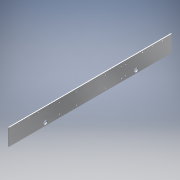
# Autodesk Inventor part: Bumper Plate
Saved by Autodesk Inventor 2019 (Build 230136000, 136)
## iProperties
Created: 2019-10-20
Part Number: Bumper Plate
Material: Aluminum 6061
Document SubType Name: Modeling
Designer: admin
Density: 2.7 g/cm^3
Appearance: Aluminum - Flat
Mass: 1233.5 g
Surface Area: 1935.72 cm^2
Volume: 456.852 cm^3
Author: admin
Autodesk Inventor part; units mm, degrees
ref_plane "YZ Plane" through (0, 0, 0) normal (1, 0, 0) x (0, 1, 0)
ref_plane "XZ Plane" through (0, 0, 0) normal (0, 1, 0) x (-1, 0, 0)
ref_plane "XY Plane" through (0, 0, 0) normal (0, 0, 1) x (1, 0, 0)
sketch "Sketch1" plane through (0, 0, 0) normal (1, 0, 0) x (0, 1, 0)
  line L0 (-50, 489.5) -> (50, 489.5)
  line L1 (50, 489.5) -> (50, -489.5)
  line L2 (50, -489.5) -> (-50, -489.5)
  line L3 (-50, -489.5) -> (-50, 489.5)
  line L4 (-50, 489.5) -> (50, -489.5) construction
  line L5 (50, 489.5) -> (-50, -489.5) construction
  point P0 (0, 0)
  dimension "d0" = 979
  dimension "d1" = 100
  constraints: 12 end point, 2 midpoint, 2 parallel, 1 horizontal, 1 perpendicular
  measures "d0" distance of L0.end L1.end
  measures "d1" distance of L0.start L0.end
extrude "Extrusion1" add sketch "Sketch1" along normal blind 5
sketch "Sketch2" plane through (5, 0, 0) normal (1, 0, 0) x (0, 0, -1)
  circle A0 centre (-270.411, -31.452) radius 12.25
  line L0 (-489.5, -50) -> (489.5, -50) projected
  line L1 (-489.5, 50) -> (-489.5, -50) projected
  circle A1 centre (274.562, -31.452) radius 12.25
  line L2 (489.5, -50) -> (489.5, 50) projected
  point P0 (0, 0)
  dimension "d4" = 24.5
  dimension "d5" = 18.548
  dimension "d8" = 219.089
  dimension "d18" = 214.938
  dimension "d19" = 24.5
  dimension "d20" = 18.548
  constraints: 2 centre point
  measures "d4" diameter of A0
  measures "d5" distance from line of L0 A0.centre
  measures "d8" distance from line of L1 A0.centre
  measures "d18" distance from line of L2 A1.centre
  measures "d19" diameter of A1
  measures "d20" distance from line of L0 A1.centre
extrude "Extrusion2" cut sketch "Sketch2" against normal through all
sketch "Sketch6" plane through (5, 0, 0) normal (1, 0, 0) x (0, 0, -1)
  circle A0 centre (274.5619, -31.452) radius 16.3 projected
  circle A1 centre (212.908, -30) radius 2.75 projected
  circle A2 centre (-124.274, -40) radius 2.75 projected
  circle A3 centre (-164.274, 40) radius 2.75 projected
  circle A4 centre (313.651, 40.5) radius 2.75 projected
  circle A5 centre (433.651, 40.5) radius 2.75 projected
  circle A6 centre (-309.5, 40.5) radius 2.75 projected
  circle A7 centre (-85, -34.5) radius 2.75 projected
  circle A8 centre (-186, 30) radius 2.75 projected
  circle A9 centre (92.5, -34.5) radius 2.75 projected
  circle A10 centre (185.908, -30) radius 2.75 projected
  circle A11 centre (185.908, 30) radius 2.75 projected
  circle A12 centre (92.5, 34.5) radius 2.75 projected
  circle A13 centre (-186, -30) radius 2.75 projected
  circle A14 centre (-85, 34.5) radius 2.75 projected
  circle A15 centre (-429.5, 40.5) radius 2.75 projected
  circle A16 centre (-369.5, 40.5) radius 2.75 projected
  circle A17 centre (373.651, 40.5) radius 2.75 projected
  circle A18 centre (-124.274, 40) radius 2.75 projected
  circle A19 centre (-154.274, -40) radius 2.75 projected
  circle A20 centre (212.908, 30) radius 2.75 projected
  circle A21 centre (148.424, 0) radius 9.8 projected
  circle A22 centre (-61.972, 12.7) radius 2.25 projected
  circle A23 centre (-87.372, 12.7) radius 2.25 projected
  circle A24 centre (-87.372, -12.7) radius 2.25 projected
  circle A25 centre (-61.972, -12.7) radius 2.25 projected
  line L0 (-19.5, -25) -> (-19.5, 25) projected
  line L1 (-19.5, 25) -> (110.5, 25) projected
  line L2 (110.5, 25) -> (110.5, -25) projected
  line L3 (110.5, -25) -> (-19.5, -25) projected
  circle A26 centre (-144.273, 0) radius 30 projected
  arc A27 (-360.3076, -42.4652) -> (-351.3744, -41.3708) centre (-355.841, -41.918) ccw projected
  arc A28 (-360.9797, -31.4275) -> (-360.3076, -42.4652) centre (-270.411, -31.452) ccw projected
  arc A29 (-351.9797, -31.4299) -> (-360.9797, -31.4275) centre (-356.4797, -31.4287) ccw projected
  arc A30 (-351.9797, -31.4299) -> (-351.3744, -41.3708) centre (-270.411, -31.452) ccw projected
  circle A31 centre (-270.411, -31.452) radius 16.3 projected
  line L4 (-469.5, 50) -> (-469.5, -50) projected
  line L5 (-469.5, -50) -> (469.5, -50) projected
  line L6 (469.5, 50) -> (469.5, -50) projected
  line L7 (-469.5, 50) -> (469.5, 50) projected
  circle A32 centre (128.424, -40) radius 2.75 projected
  circle A33 centre (128.424, 40) radius 2.75 projected
  circle A34 centre (168.424, 40) radius 2.75 projected
  circle A35 centre (158.424, -40) radius 2.75 projected
  point P0 (0, 0)
extrude "Extrusion4" cut sketch "Sketch6" against normal blind 10 contours A1 | A4 | A5 | A6 | A7 | A8 | A9 | A10 | A11 | A12 | A13 | A14 | A15 | A16 | A17 | A20
equation "\"d20\" = d5"
body "Solid1"
